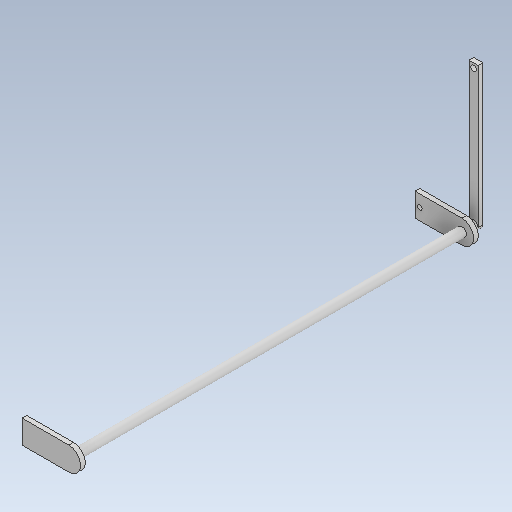
# Autodesk Inventor part: LenkungHinten
Saved by Autodesk Inventor 2020 (Build 240168000, 168)
## iProperties
Created: 2020-02-20
Part Number: LenkungHinten
Material: Generisch
Document SubType Name: Modeling
Designer: Stefan
Density: 1 g/cm^3
Appearance: Vorgabe
Mass: 430.069 g
Surface Area: 998.766 cm^2
Volume: 430.069 cm^3
Author: Stefan
Autodesk Inventor part; units mm, degrees
ref_plane "YZ Plane" through (0, 0, 0) normal (1, 0, 0) x (0, 1, 0)
ref_plane "XZ Plane" through (0, 0, 0) normal (0, 1, 0) x (-1, 0, 0)
ref_plane "XY Plane" through (0, 0, 0) normal (0, 0, 1) x (1, 0, 0)
sketch "Skizze1" plane through (0, 0, 0) normal (0, 0, 1) x (1, 0, 0)
  circle A0 centre (0, 0) radius 9.75
  dimension "d0" = 19.5
  constraints: 1 centre point, 1 coincident
  measures "d0" diameter of A0
extrude "Extrusion1" add sketch "Skizze1" along normal blind 830
sketch "Skizze4" plane through (0, 0, 830) normal (0, 0, 1) x (1, 0, 0)
  arc A0 (0, -25) -> (0, 25) centre (0, 0) ccw
  line L0 (0, 0) -> (0, -25) construction
  line L1 (0, 0) -> (0, 27.5151) construction
  line L2 (0, 25) -> (-100, 25)
  line L3 (-100, 25) -> (-100, -25)
  line L4 (-100, -25) -> (0, -25)
  point P0 (0, 25)
  dimension "d9" = 180
  dimension "d10" = 100
  dimension "d11" = 50
  dimension "d12" = 25
  constraints: 10 end point, 2 perpendicular, 2 point on circle, 1 centre point, 1 coincident, 1 horizontal, 1 point on line
  measures "d9" angle of L0 L1
  measures "d10" distance of L2.start L2.end
  measures "d11" distance of L2.end L3.end
  measures "d12" distance of point (0, 0) A0.end
extrude "Extrusion4" add sketch "Skizze4" along normal blind 10
sketch "Skizze5" plane through (0, 0, 0) normal (0, 0, -1) x (-1, 0, 0)
  arc A0 (0, 25) -> (0, -25) centre (0, 0) ccw
  line L0 (0, 25) -> (100, 25)
  line L1 (100, 25) -> (100, -25)
  line L2 (100, -25) -> (0, -25)
  dimension "d15" = 25
  dimension "d16" = 0
  dimension "d17" = 0
  dimension "d18" = 100
  dimension "d19" = 50
  dimension "d20" = 90
  constraints: 6 end point, 3 point on circle, 2 perpendicular, 1 centre point, 1 coincident, 1 horizontal
  measures "d15" radius of A0
  measures "d16" horizontal distance of point (0, 0) L0.start
  measures "d17" horizontal distance of point (0, 0) A0.end
  measures "d18" distance of L0.start L0.end
  measures "d19" distance of L0.end L1.end
  measures "d20" angle of L0 L1
extrude "Extrusion5" add sketch "Skizze5" along normal blind 10
sketch "Skizze6" plane through (0, 0, 0) normal (0, 0, 1) x (1, 0, 0)
  circle A0 centre (-90, 0) radius 5
  line L0 (-100, 25) -> (0, 25) projected
  line L1 (-100, -25) -> (-100, 25) projected
  point P0 (0, 0)
  dimension "d23" = 10
  dimension "d24" = 25
  dimension "d25" = 10
  constraints: 1 centre point
  measures "d23" diameter of A0
  measures "d24" distance from line of L0 A0.centre
  measures "d25" distance from line of L1 A0.centre
extrude "Extrusion6" cut sketch "Skizze6" against normal up to surface (10 mm away)
sketch "Skizze7" plane through (0, 0, -10) normal (0, 0, -1) x (-1, 0, 0)
  circle A0 centre (0, 0) radius 9.75
  dimension "d28" = 19.5
  constraints: 1 centre point, 1 coincident
  measures "d28" diameter of A0
extrude "Extrusion7" add sketch "Skizze7" along normal blind 15
sketch "Skizze8" plane through (0, 0, -25) normal (0, 0, -1) x (-1, 0, 0)
  line L0 (9.75, 0) -> (-9.75, 0)
  line L1 (-9.75, 0) -> (-9.75, 300)
  line L2 (-9.75, 300) -> (9.75, 300)
  line L3 (9.75, 300) -> (9.75, 0)
  circle A0 centre (0, 0) radius 9.75
  circle A1 centre (0, 0) radius 9.75
  dimension "d31" = 300
  dimension "d32" = 19.5
  dimension "d33" = 9.75
  dimension "d34" = 0
  dimension "d35" = 19.5
  constraints: 8 end point, 2 coincident, 2 parallel, 1 centre point, 1 horizontal, 1 perpendicular, 3 other
  measures "d31" distance of L0.end L1.end
  measures "d32" distance of L0.start L0.end
  measures "d33" distance from line of point (0, 0) L3
  measures "d34" distance from line of point (0, 0) L0
  measures "d35" diameter of A1
extrude "Extrusion8" add sketch "Skizze8" along normal blind 10
sketch "Skizze9" plane through (0, 0, -25) normal (0, 0, 1) x (1, 0, 0)
  circle A0 centre (0, 290) radius 6
  line L0 (9.75, 300) -> (9.75, 0) projected
  line L1 (-9.75, 300) -> (9.75, 300) projected
  point P0 (0, 0)
  dimension "d38" = 12
  dimension "d39" = 9.75
  dimension "d40" = 10
  constraints: 1 centre point
  measures "d38" diameter of A0
  measures "d39" distance from line of L0 A0.centre
  measures "d40" distance from line of L1 A0.centre
extrude "Extrusion9" cut sketch "Skizze9" against normal up to surface (10 mm away)
